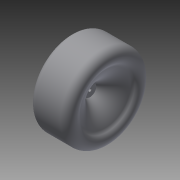
# Autodesk Inventor part: kolo
Saved by Autodesk Inventor 2015 (Build 190159000, 159)
## iProperties
Created: 2015-01-01
Part Number: kolo
Material: Generic
Document SubType Name: Modeling
Designer: Turboslimak
Density: 1 g/cm^3
Appearance: Default
Author: Turboslimak
Autodesk Inventor part; units mm, degrees
ref_plane "YZ Plane" through (0, 0, 0) normal (1, 0, 0) x (0, 1, 0)
ref_plane "XZ Plane" through (0, 0, 0) normal (0, 1, 0) x (-1, 0, 0)
ref_plane "XY Plane" through (0, 0, 0) normal (0, 0, 1) x (1, 0, 0)
sketch "Sketch1" plane through (0, 0, 0) normal (0, 1, 0) x (-1, 0, 0)
  line L0 (28, -60) -> (-28, -60)
  line L1 (10, 0) -> (10, -9)
  line L2 (10, -9) -> (-2.5336, -34.9761)
  arc A0 (-2.5336, -34.9761) -> (1, -40) centre (0.6326, -36.5038) ccw
  line L3 (26, -40) -> (26, -44)
  line L4 (26, -44) -> (28, -44)
  line L5 (28, -44) -> (28, -60)
  line L6 (26, -40) -> (1, -40)
  line L7 (-28, -39) -> (-23, -39)
  arc A1 (0, -9) -> (-23, -39) centre (26.2528, -52.9438) ccw
  line L8 (-28, -39) -> (-28, -60)
  line L9 (10, 0) -> (0, 0)
  line L10 (0, -9) -> (0, 0)
  line L11 (0, 0) -> (10, 0)
  line L12 (10, -9) -> (10, 0)
  line L13 (0, 0) -> (10, 0)
  line L14 (0, 0) -> (0, -9)
  dimension "d9" = 4
  dimension "d12" = 5
  constraints: 30 end point, 5 point on circle, 4 collinear, 2 centre point, 1 coincident, 1 tangent, 1 vertical
  measures "d9" distance of L3.start L3.end
  measures "d12" distance of L7.start L7.end
revolve "Revolution1" add sketch "Sketch1" angle 360 about axis through (0, 0, 0) along (-1, 0, 0)
sketch "Sketch2" plane through (0, 0, 0) normal (1, 0, 0) x (0, 0, -1)
  circle A0 centre (0, 0) radius 2.1
  dimension "d16" = 4.2
  constraints: 1 centre point, 1 coincident
  measures "d16" diameter of A0
extrude "Extrusion1" cut sketch "Sketch2" against normal blind 10
fillet "Fillet1" radius 10 1 edges at (-28, 0, 44)
fillet "Fillet2" radius 9.25 1 edges at (-28, 0, 60)
fillet "Fillet3" radius 11.25 2 edges at (28, 0, 39) (28, 0, 60)
fillet "Fillet4" radius 10.25 1 edges at (23, 0, 39)
body "Solid1"
